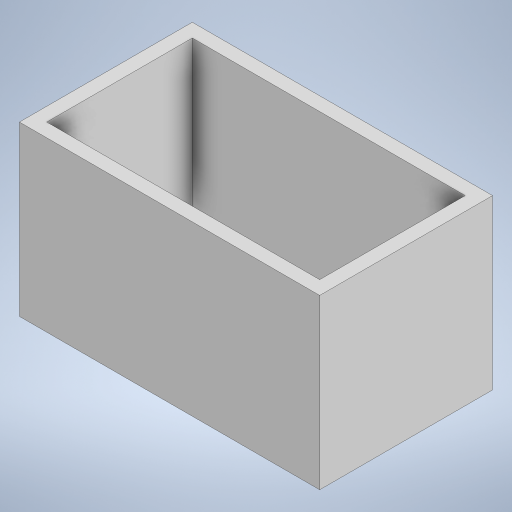
# Autodesk Inventor part: 전체 하우징
Saved by Autodesk Inventor 2023 (Build 270158000, 158)
## iProperties
Created: 2022-08-25
Part Number: 전체 하우징
Material: 일반
Document SubType Name: Modeling
Designer: user
Density: 1 g/cm^3
Appearance: 기본값
Author: user
Autodesk Inventor part; units mm, degrees
ref_plane "YZ Plane" through (0, 0, 0) normal (1, 0, 0) x (0, 1, 0)
ref_plane "XZ Plane" through (0, 0, 0) normal (0, 1, 0) x (-1, 0, 0)
ref_plane "XY Plane" through (0, 0, 0) normal (0, 0, 1) x (1, 0, 0)
sketch "스케치1" plane through (0, 0, 0) normal (0, 1, 0) x (-1, 0, 0)
  line L0 (30, 16) -> (-30, 16)
  line L1 (-30, 16) -> (-30, -16)
  line L2 (-30, -16) -> (30, -16)
  line L3 (30, 16) -> (-30, -16) construction
  line L4 (-30, 16) -> (30, -16) construction
  line L5 (30, -16) -> (30, 16)
  line L6 (33, 19) -> (-33, 19)
  line L7 (-33, 19) -> (-33, -19)
  line L8 (-33, -19) -> (33, -19)
  line L9 (33, -19) -> (33, 19)
  point P0 (0, 0)
  dimension "d0" = 60
  dimension "d1" = 32
  dimension "d6" = 3
  constraints: 20 end point, 2 midpoint, 2 parallel, 2 perpendicular, 1 horizontal, 1 vertical, 3 other
  measures "d0" distance of L2.end L1.end
  measures "d1" distance of L1.end L0.end
  measures "d6" distance between parallel lines of L5 L9
extrude "돌출1" add sketch "스케치1" against normal blind 3 contours L5 L2 L1 L0 | L9 L8 L7 L6
extrude "돌출2" add sketch "스케치1" along normal blind 34
sketch "스케치2" plane through (0, 0, 0) normal (0, 1, 0) x (1, 0, 0)
  circle A0 centre (-20.5, -6) radius 1
  circle A1 centre (-14.5, -6) radius 1
  line L0 (-30, 16) -> (30, 16) projected
  line L1 (-30, -16) -> (-30, 16) projected
  point P0 (0, 0)
  dimension "d11" = 2
  dimension "d12" = 2
  dimension "d13" = 6
  dimension "d14" = 22
  dimension "d15" = 9.5
  constraints: 2 centre point, 1 horizontal alignment
  measures "d11" diameter of A0
  measures "d12" diameter of A1
  measures "d13" distance of A1.centre A0.centre
  measures "d14" distance from line of L0 A0.centre
  measures "d15" distance from line of L1 A0.centre
extrude "돌출3" cut sketch "스케치2" against normal blind 10
sketch "스케치3" plane through (0, 0, 0) normal (0, 1, 0) x (1, 0, 0)
  line L0 (30, -16) -> (-30, -16) projected
  line L1 (-2.1, -16) -> (2.2, -16)
  line L2 (2.2, -16) -> (2.2, -4)
  line L3 (2.2, -4) -> (-2.1, -4)
  line L4 (-2.1, -4) -> (-2.1, -16)
  line L5 (25.7, -4) -> (30, -4)
  line L6 (30, -4) -> (30, -16)
  line L7 (30, -16) -> (25.7, -16)
  line L8 (25.7, -16) -> (25.7, -4)
  circle A0 centre (0.05, -10) radius 1
  circle A1 centre (28.25, -10) radius 1
  point P0 (0, 0)
  point P1 (0.05, -4)
  point P2 (2.2, -10)
  dimension "d18" = 12
  dimension "d19" = 23.5
  dimension "d20" = 32.1
  dimension "d21" = 2
  dimension "d22" = 2
  dimension "d23" = 28.2
  constraints: 16 end point, 4 parallel, 3 point on line, 2 centre point, 2 horizontal, 2 horizontal alignment, 2 midpoint, 2 perpendicular, 1 collinear, 1 vertical alignment
  measures "d18" distance of L3.end L1.start
  measures "d19" distance between parallel lines of L8 L2
  measures "d20" distance between parallel lines of L6 L4
  measures "d21" diameter of A0
  measures "d22" diameter of A1
  measures "d23" distance of A1.centre A0.centre
extrude "돌출4" add sketch "스케치3" along normal blind 19
sketch "스케치4" plane through (-2.1, 0, 4) normal (-1, 0, 0) x (0, 0, 1)
  line L0 (0, 0) -> (12, 0) projected
  line L1 (9, 0) -> (3, 0)
  line L2 (3, 0) -> (3, 7)
  line L3 (6, 10) -> (6, 10)
  line L4 (9, 7) -> (9, 0)
  line L5 (3, 7) -> (6, 10)
  line L6 (6, 10) -> (9, 7)
  point P0 (-4, 0)
  point P1 (3, 10)
  point P2 (9, 10)
  point P3 (6, 0)
  point P4 (6, 10)
  point P5 (3, 0)
  dimension "d26" = 6
  dimension "d27" = 10
  dimension "d28" = 3
  dimension "d29" = 3
  dimension "d30" = 3
  dimension "d31" = 3
  constraints: 12 end point, 5 point on line, 2 midpoint, 2 parallel, 1 horizontal, 1 perpendicular
  measures "d26" distance of point (3, 10) point (9, 10)
  measures "d27" distance of L1.end point (3, 10)
  measures "d28" distance of L2.end point (3, 10)
  measures "d29" distance of L3.start point (3, 10)
  measures "d30" distance of L3.end point (9, 10)
  measures "d31" distance of L4.start point (9, 10)
extrude "돌출5" cut sketch "스케치4" against normal up to surface (4.3 mm away)
sketch "스케치5" plane through (25.7, 0, 4) normal (-1, 0, 0) x (0, 0, 1)
  line L0 (0, 13.3063) -> (8, 5.3063)
  line L1 (8, 5.3063) -> (8, 0)
  line L2 (7, 19) -> (7, 0) projected
  line L3 (0, 0) -> (-20, 0) projected
  line L4 (8, 0) -> (0, 0)
  line L5 (0, 0) -> (0, 13.3063)
  point P0 (-4, 0)
  dimension "d34" = 45
  dimension "d35" = 8
  constraints: 8 end point, 2 perpendicular, 1 parallel
  measures "d34" angle of L5 L0
  measures "d35" distance between parallel lines of L5 L1
extrude "돌출6" cut sketch "스케치5" against normal up to surface (4.3 mm away)
equation "\"d29\" = d28"
equation "\"d30\" = d28"
equation "\"d31\" = d30"
